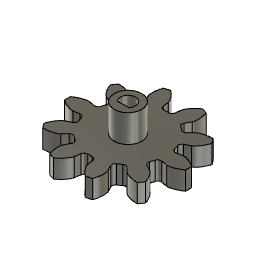
gear motor (Autodesk Fusion 360 design; units mm, degrees)
description: Spur Gear; Module: 2.2; Num Teeth: 10; Pressure Angle: 20.0; Backlash: 0.00 mm
Autodesk Fusion 360 part; units mm, degrees
(part 1 of 2)
sketch "gear motor 1" plane through (0, 0, 0) normal (0, 0, 1) x (1, 0, 0) in component "gear motor (1)"
  circle A0 centre (0, 0) radius 8.3092
  circle A1 centre (0, 0) radius 1.65
extrude "Extrude1" add sketch "gear motor 1" along normal blind 4 in component "gear motor (1)"
sketch "gear motor 2" plane through (0, 0, 0) normal (0, 0, 1) x (1, 0, 0) in component "gear motor (1)"
  spline S0 degree 5 poles (10.1841, -1.769) (10.1925, -1.7704) (10.2094, -1.7731) (10.2348, -1.7761) (10.2689, -1.7786) (10.3116, -1.7794) (10.3546, -1.7786) (10.3977, -1.7768) (10.4408, -1.7744) (10.484, -1.7717) (10.5273, -1.7685) (10.5706, -1.7648) (10.614, -1.7604) (10.6574, -1.7552) (10.7008, -1.7492) (10.7443, -1.7425) (10.7879, -1.7351) (10.8314, -1.7271) (10.875, -1.7187) (10.9186, -1.7098) (10.9622, -1.7005) (11.0058, -1.6907) (11.0494, -1.6804) (11.0931, -1.6695) (11.1367, -1.6581) (11.1803, -1.6463) (11.2239, -1.6339) (11.2675, -1.6212) (11.3111, -1.608) (11.3547, -1.5943) (11.3982, -1.5802) (11.4418, -1.5657) (11.4853, -1.5508) (11.5288, -1.5355) (11.5722, -1.5197) (11.6157, -1.5035) (11.6591, -1.4869) (11.7024, -1.4699) (11.7457, -1.4525) (11.789, -1.4347) (11.8323, -1.4166) (11.8755, -1.398) (11.9187, -1.3791) (11.9618, -1.3598) (12.0049, -1.3401) (12.0479, -1.32) (12.0909, -1.2996) (12.1338, -1.2787) (12.1766, -1.2576) (12.2194, -1.236) (12.2622, -1.2141) (12.3049, -1.1919) (12.3475, -1.1693) (12.3901, -1.1463) (12.4325, -1.123) (12.475, -1.0994) (12.5173, -1.0754) (12.5596, -1.0511) (12.6018, -1.0264) (12.6439, -1.0014) (12.686, -0.976) (12.728, -0.9503) (12.7699, -0.9243) (12.8117, -0.898) (12.8535, -0.8713) (12.8951, -0.8443) (12.9367, -0.817) (12.9782, -0.7893) (13.0195, -0.7613) (13.0608, -0.7331) (13.102, -0.7045) (13.1349, -0.6813) (13.1596, -0.6638) (13.176, -0.6521) (13.1842, -0.6462) knots 0 0 0 0 0 0 0.01428571 0.02857143 0.04285714 0.05714286 0.07142857 0.08571429 0.1 0.11428571 0.12857143 0.14285714 0.15714286 0.17142857 0.18571429 0.2 0.21428571 0.22857143 0.24285714 0.25714286 0.27142857 0.28571429 0.3 0.31428571 0.32857143 0.34285714 0.35714286 0.37142857 0.38571429 0.4 0.41428571 0.42857143 0.44285714 0.45714286 0.47142857 0.48571429 0.5 0.51428571 0.52857143 0.54285714 0.55714286 0.57142857 0.58571429 0.6 0.61428571 0.62857143 0.64285714 0.65714286 0.67142857 0.68571429 0.7 0.71428571 0.72857143 0.74285714 0.75714286 0.77142857 0.78571429 0.8 0.81428571 0.82857143 0.84285714 0.85714286 0.87142857 0.88571429 0.9 0.91428571 0.92857143 0.94285714 0.95714286 0.97142857 0.98571429 1 1 1 1 1 1
  spline S1 degree 5 poles (10.1841, 1.769) (10.1925, 1.7704) (10.2094, 1.7731) (10.2348, 1.7761) (10.2689, 1.7786) (10.3116, 1.7794) (10.3546, 1.7786) (10.3977, 1.7768) (10.4408, 1.7744) (10.484, 1.7717) (10.5273, 1.7685) (10.5706, 1.7648) (10.614, 1.7604) (10.6574, 1.7552) (10.7008, 1.7492) (10.7443, 1.7425) (10.7879, 1.7351) (10.8314, 1.7271) (10.875, 1.7187) (10.9186, 1.7098) (10.9622, 1.7005) (11.0058, 1.6907) (11.0494, 1.6804) (11.0931, 1.6695) (11.1367, 1.6581) (11.1803, 1.6463) (11.2239, 1.6339) (11.2675, 1.6212) (11.3111, 1.608) (11.3547, 1.5943) (11.3982, 1.5802) (11.4418, 1.5657) (11.4853, 1.5508) (11.5288, 1.5355) (11.5722, 1.5197) (11.6157, 1.5035) (11.6591, 1.4869) (11.7024, 1.4699) (11.7457, 1.4525) (11.789, 1.4347) (11.8323, 1.4166) (11.8755, 1.398) (11.9187, 1.3791) (11.9618, 1.3598) (12.0049, 1.3401) (12.0479, 1.32) (12.0909, 1.2996) (12.1338, 1.2787) (12.1766, 1.2576) (12.2194, 1.236) (12.2622, 1.2141) (12.3049, 1.1919) (12.3475, 1.1693) (12.3901, 1.1463) (12.4325, 1.123) (12.475, 1.0994) (12.5173, 1.0754) (12.5596, 1.0511) (12.6018, 1.0264) (12.6439, 1.0014) (12.686, 0.976) (12.728, 0.9503) (12.7699, 0.9243) (12.8117, 0.898) (12.8535, 0.8713) (12.8951, 0.8443) (12.9367, 0.817) (12.9782, 0.7893) (13.0195, 0.7613) (13.0608, 0.7331) (13.102, 0.7045) (13.1349, 0.6813) (13.1596, 0.6638) (13.176, 0.6521) (13.1842, 0.6462) knots 0 0 0 0 0 0 0.01428571 0.02857143 0.04285714 0.05714286 0.07142857 0.08571429 0.1 0.11428571 0.12857143 0.14285714 0.15714286 0.17142857 0.18571429 0.2 0.21428571 0.22857143 0.24285714 0.25714286 0.27142857 0.28571429 0.3 0.31428571 0.32857143 0.34285714 0.35714286 0.37142857 0.38571429 0.4 0.41428571 0.42857143 0.44285714 0.45714286 0.47142857 0.48571429 0.5 0.51428571 0.52857143 0.54285714 0.55714286 0.57142857 0.58571429 0.6 0.61428571 0.62857143 0.64285714 0.65714286 0.67142857 0.68571429 0.7 0.71428571 0.72857143 0.74285714 0.75714286 0.77142857 0.78571429 0.8 0.81428571 0.82857143 0.84285714 0.85714286 0.87142857 0.88571429 0.9 0.91428571 0.92857143 0.94285714 0.95714286 0.97142857 0.98571429 1 1 1 1 1 1
  arc A0 (13.1842, -0.6462) -> (13.1842, 0.6462) centre (0, 0) ccw
  line L0 (8.1768, -1.422) -> (10.1841, -1.769)
  line L1 (8.1768, 1.422) -> (10.1841, 1.769)
  line L2 (8.1768, -1.422) -> (8.1768, 1.422)
  point P0 (10.3903, -1.777)
  point P1 (10.6003, -1.7617)
  point P2 (10.8126, -1.7305)
  point P3 (11.0266, -1.6857)
  point P4 (11.2419, -1.6286)
  point P5 (11.4581, -1.5601)
  point P6 (11.6748, -1.4807)
  point P7 (11.8918, -1.3908)
  point P8 (12.1088, -1.2908)
  point P9 (12.3254, -1.1809)
  point P10 (12.5416, -1.0614)
  point P11 (12.7569, -0.9323)
  point P12 (12.9712, -0.7939)
  point P13 (10.3903, 1.777)
  point P14 (10.6003, 1.7617)
  point P15 (10.8126, 1.7305)
  point P16 (11.0266, 1.6857)
  point P17 (11.2419, 1.6286)
  point P18 (11.4581, 1.5601)
  point P19 (11.6748, 1.4807)
  point P20 (11.8918, 1.3908)
  point P21 (12.1088, 1.2908)
  point P22 (12.3254, 1.1809)
  point P23 (12.5416, 1.0614)
  point P24 (12.7569, 0.9323)
  point P25 (12.9712, 0.7939)
extrude "Extrude2" add sketch "gear motor 2" along normal blind 4 in component "gear motor (1)"
fillet "Fillet1" radius 0.75 2 edges at (8.1863, -1.4237, 2) (8.1863, 1.4237, 2) in component "gear motor (1)"
pattern_circular "C-Pattern1" count 10 over 360 about axis through (0, 0, 0) along (0, 0, 1) of "Extrude2", "Fillet1" in component "gear motor (1)"
sketch "gear motor 3" plane through (0, 0, 0) normal (0, 0, 1) x (1, 0, 0) in component "gear motor (1)"
  circle A0 centre (0, 0) radius 11 construction
mesh "Mesh1" [no effect] in component "gear motor (1)"
sketch "gear motor detailed cut" plane through (0, 0, 4) normal (0, 0, 1) x (-1, 0, 0) in component "gear motor (1)"
  arc A0 (-7.7368, 3.0305) -> (-8.0405, 2.0959) centre (0, 0) ccw
  arc A1 (-8.894, 1.546) -> (-8.0405, 2.0959) centre (-8.7663, 2.285) ccw
  line L0 (-8.894, 1.546) -> (-10.1841, 1.769)
  spline S0 degree 5 poles (-10.1841, 1.769) (-10.1925, 1.7704) (-10.2094, 1.7731) (-10.2348, 1.7761) (-10.2689, 1.7786) (-10.3116, 1.7794) (-10.3546, 1.7786) (-10.3977, 1.7768) (-10.4408, 1.7744) (-10.484, 1.7717) (-10.5273, 1.7685) (-10.5706, 1.7648) (-10.614, 1.7604) (-10.6574, 1.7552) (-10.7008, 1.7492) (-10.7443, 1.7425) (-10.7879, 1.7351) (-10.8314, 1.7271) (-10.875, 1.7187) (-10.9186, 1.7098) (-10.9622, 1.7005) (-11.0058, 1.6907) (-11.0494, 1.6804) (-11.0931, 1.6695) (-11.1367, 1.6581) (-11.1803, 1.6463) (-11.2239, 1.6339) (-11.2675, 1.6212) (-11.3111, 1.608) (-11.3547, 1.5943) (-11.3982, 1.5802) (-11.4418, 1.5657) (-11.4853, 1.5508) (-11.5288, 1.5355) (-11.5722, 1.5197) (-11.6157, 1.5035) (-11.6591, 1.4869) (-11.7024, 1.4699) (-11.7457, 1.4525) (-11.789, 1.4347) (-11.8323, 1.4166) (-11.8755, 1.398) (-11.9187, 1.3791) (-11.9618, 1.3598) (-12.0049, 1.3401) (-12.0479, 1.32) (-12.0909, 1.2996) (-12.1338, 1.2787) (-12.1766, 1.2576) (-12.2194, 1.236) (-12.2622, 1.2141) (-12.3049, 1.1919) (-12.3475, 1.1693) (-12.3901, 1.1463) (-12.4325, 1.123) (-12.475, 1.0994) (-12.5173, 1.0754) (-12.5596, 1.0511) (-12.6018, 1.0264) (-12.6439, 1.0014) (-12.686, 0.976) (-12.728, 0.9503) (-12.7699, 0.9243) (-12.8117, 0.898) (-12.8535, 0.8713) (-12.8951, 0.8443) (-12.9367, 0.817) (-12.9782, 0.7893) (-13.0195, 0.7613) (-13.0608, 0.7331) (-13.102, 0.7045) (-13.1349, 0.6813) (-13.1596, 0.6638) (-13.176, 0.6521) (-13.1842, 0.6462) knots 0 0 0 0 0 0 0.01428571 0.02857143 0.04285714 0.05714286 0.07142857 0.08571429 0.1 0.11428571 0.12857143 0.14285714 0.15714286 0.17142857 0.18571429 0.2 0.21428571 0.22857143 0.24285714 0.25714286 0.27142857 0.28571429 0.3 0.31428571 0.32857143 0.34285714 0.35714286 0.37142857 0.38571429 0.4 0.41428571 0.42857143 0.44285714 0.45714286 0.47142857 0.48571429 0.5 0.51428571 0.52857143 0.54285714 0.55714286 0.57142857 0.58571429 0.6 0.61428571 0.62857143 0.64285714 0.65714286 0.67142857 0.68571429 0.7 0.71428571 0.72857143 0.74285714 0.75714286 0.77142857 0.78571429 0.8 0.81428571 0.82857143 0.84285714 0.85714286 0.87142857 0.88571429 0.9 0.91428571 0.92857143 0.94285714 0.95714286 0.97142857 0.98571429 1 1 1 1 1 1
  arc A2 (-13.1842, 0.6462) -> (-13.1842, -0.6462) centre (0, 0) ccw
  spline S1 degree 5 poles (-13.1842, -0.6462) (-13.176, -0.6521) (-13.1596, -0.6638) (-13.1349, -0.6813) (-13.102, -0.7045) (-13.0608, -0.7331) (-13.0195, -0.7613) (-12.9782, -0.7893) (-12.9367, -0.817) (-12.8951, -0.8443) (-12.8535, -0.8713) (-12.8117, -0.898) (-12.7699, -0.9243) (-12.728, -0.9503) (-12.686, -0.976) (-12.6439, -1.0014) (-12.6018, -1.0264) (-12.5596, -1.0511) (-12.5173, -1.0754) (-12.475, -1.0994) (-12.4325, -1.123) (-12.3901, -1.1463) (-12.3475, -1.1693) (-12.3049, -1.1919) (-12.2622, -1.2141) (-12.2194, -1.236) (-12.1766, -1.2576) (-12.1338, -1.2787) (-12.0909, -1.2996) (-12.0479, -1.32) (-12.0049, -1.3401) (-11.9618, -1.3598) (-11.9187, -1.3791) (-11.8755, -1.398) (-11.8323, -1.4166) (-11.789, -1.4347) (-11.7457, -1.4525) (-11.7024, -1.4699) (-11.6591, -1.4869) (-11.6157, -1.5035) (-11.5722, -1.5197) (-11.5288, -1.5355) (-11.4853, -1.5508) (-11.4418, -1.5657) (-11.3982, -1.5802) (-11.3547, -1.5943) (-11.3111, -1.608) (-11.2675, -1.6212) (-11.2239, -1.6339) (-11.1803, -1.6463) (-11.1367, -1.6581) (-11.0931, -1.6695) (-11.0494, -1.6804) (-11.0058, -1.6907) (-10.9622, -1.7005) (-10.9186, -1.7098) (-10.875, -1.7187) (-10.8314, -1.7271) (-10.7879, -1.7351) (-10.7443, -1.7425) (-10.7008, -1.7492) (-10.6574, -1.7552) (-10.614, -1.7604) (-10.5706, -1.7648) (-10.5273, -1.7685) (-10.484, -1.7717) (-10.4408, -1.7744) (-10.3977, -1.7768) (-10.3546, -1.7786) (-10.3116, -1.7794) (-10.2689, -1.7786) (-10.2348, -1.7761) (-10.2094, -1.7731) (-10.1925, -1.7704) (-10.1841, -1.769) knots -1 -1 -1 -1 -1 -1 -0.98571429 -0.97142857 -0.95714286 -0.94285714 -0.92857143 -0.91428571 -0.9 -0.88571429 -0.87142857 -0.85714286 -0.84285714 -0.82857143 -0.81428571 -0.8 -0.78571429 -0.77142857 -0.75714286 -0.74285714 -0.72857143 -0.71428571 -0.7 -0.68571429 -0.67142857 -0.65714286 -0.64285714 -0.62857143 -0.61428571 -0.6 -0.58571429 -0.57142857 -0.55714286 -0.54285714 -0.52857143 -0.51428571 -0.5 -0.48571429 -0.47142857 -0.45714286 -0.44285714 -0.42857143 -0.41428571 -0.4 -0.38571429 -0.37142857 -0.35714286 -0.34285714 -0.32857143 -0.31428571 -0.3 -0.28571429 -0.27142857 -0.25714286 -0.24285714 -0.22857143 -0.21428571 -0.2 -0.18571429 -0.17142857 -0.15714286 -0.14285714 -0.12857143 -0.11428571 -0.1 -0.08571429 -0.07142857 -0.05714286 -0.04285714 -0.02857143 -0.01428571 0 0 0 0 0 0
  line L1 (-10.1841, -1.769) -> (-8.894, -1.546)
  arc A3 (-8.0405, -2.0959) -> (-8.894, -1.546) centre (-8.7663, -2.285) ccw
  arc A4 (-8.0405, -2.0959) -> (-7.7368, -3.0305) centre (0, 0) ccw
  arc A5 (-8.1041, -3.977) -> (-7.7368, -3.0305) centre (-8.4352, -3.3041) ccw
  line L2 (-8.1041, -3.977) -> (-9.2789, -4.5549)
  spline S2 degree 5 poles (-9.2789, -4.5549) (-9.2866, -4.5587) (-9.3018, -4.5665) (-9.3241, -4.579) (-9.3531, -4.597) (-9.3882, -4.6215) (-9.4225, -4.6474) (-9.4563, -4.6742) (-9.4898, -4.7014) (-9.5231, -4.7291) (-9.5563, -4.757) (-9.5891, -4.7855) (-9.6216, -4.8145) (-9.6537, -4.8442) (-9.6853, -4.8746) (-9.7166, -4.9057) (-9.7474, -4.9373) (-9.778, -4.9693) (-9.8083, -5.0017) (-9.8384, -5.0345) (-9.8682, -5.0677) (-9.8977, -5.1013) (-9.9269, -5.1353) (-9.9558, -5.1697) (-9.9844, -5.2045) (-10.0127, -5.2397) (-10.0407, -5.2754) (-10.0685, -5.3113) (-10.096, -5.3476) (-10.1232, -5.3843) (-10.1502, -5.4213) (-10.1769, -5.4586) (-10.2033, -5.4962) (-10.2295, -5.5342) (-10.2554, -5.5725) (-10.281, -5.6111) (-10.3064, -5.6501) (-10.3314, -5.6893) (-10.3563, -5.7289) (-10.3809, -5.7687) (-10.4052, -5.8088) (-10.4292, -5.8492) (-10.453, -5.8899) (-10.4765, -5.9309) (-10.4998, -5.9721) (-10.5228, -6.0137) (-10.5456, -6.0555) (-10.5681, -6.0975) (-10.5903, -6.1399) (-10.6123, -6.1824) (-10.634, -6.2253) (-10.6554, -6.2684) (-10.6766, -6.3117) (-10.6976, -6.3553) (-10.7182, -6.3991) (-10.7387, -6.4432) (-10.7588, -6.4875) (-10.7787, -6.532) (-10.7984, -6.5768) (-10.8178, -6.6218) (-10.8369, -6.667) (-10.8557, -6.7125) (-10.8744, -6.7582) (-10.8927, -6.8041) (-10.9108, -6.8502) (-10.9286, -6.8965) (-10.9462, -6.943) (-10.9635, -6.9898) (-10.9805, -7.0367) (-10.9973, -7.0839) (-11.0139, -7.1313) (-11.0269, -7.1693) (-11.0365, -7.198) (-11.0429, -7.2171) (-11.0461, -7.2267) knots 0 0 0 0 0 0 0.01428571 0.02857143 0.04285714 0.05714286 0.07142857 0.08571429 0.1 0.11428571 0.12857143 0.14285714 0.15714286 0.17142857 0.18571429 0.2 0.21428571 0.22857143 0.24285714 0.25714286 0.27142857 0.28571429 0.3 0.31428571 0.32857143 0.34285714 0.35714286 0.37142857 0.38571429 0.4 0.41428571 0.42857143 0.44285714 0.45714286 0.47142857 0.48571429 0.5 0.51428571 0.52857143 0.54285714 0.55714286 0.57142857 0.58571429 0.6 0.61428571 0.62857143 0.64285714 0.65714286 0.67142857 0.68571429 0.7 0.71428571 0.72857143 0.74285714 0.75714286 0.77142857 0.78571429 0.8 0.81428571 0.82857143 0.84285714 0.85714286 0.87142857 0.88571429 0.9 0.91428571 0.92857143 0.94285714 0.95714286 0.97142857 0.98571429 1 1 1 1 1 1
  arc A6 (-11.0461, -7.2267) -> (-10.2864, -8.2723) centre (0, 0) ccw
  spline S3 degree 5 poles (-10.2864, -8.2723) (-10.2763, -8.2722) (-10.2561, -8.2721) (-10.2259, -8.2717) (-10.1857, -8.2711) (-10.1356, -8.27) (-10.0855, -8.2686) (-10.0356, -8.2669) (-9.9858, -8.2649) (-9.9361, -8.2626) (-9.8865, -8.26) (-9.8371, -8.257) (-9.7878, -8.2537) (-9.7386, -8.2502) (-9.6895, -8.2463) (-9.6406, -8.242) (-9.5918, -8.2375) (-9.5431, -8.2327) (-9.4946, -8.2275) (-9.4463, -8.222) (-9.398, -8.2162) (-9.35, -8.2101) (-9.302, -8.2037) (-9.2543, -8.1969) (-9.2067, -8.1898) (-9.1592, -8.1824) (-9.1119, -8.1746) (-9.0648, -8.1666) (-9.0179, -8.1582) (-8.9711, -8.1495) (-8.9245, -8.1404) (-8.878, -8.131) (-8.8318, -8.1213) (-8.7858, -8.1113) (-8.7399, -8.1009) (-8.6942, -8.0902) (-8.6487, -8.0791) (-8.6035, -8.0677) (-8.5584, -8.056) (-8.5135, -8.0439) (-8.4689, -8.0314) (-8.4244, -8.0187) (-8.3802, -8.0055) (-8.3363, -7.992) (-8.2925, -7.9781) (-8.249, -7.9639) (-8.2057, -7.9494) (-8.1627, -7.9344) (-8.1199, -7.9191) (-8.0774, -7.9035) (-8.0351, -7.8874) (-7.9932, -7.871) (-7.9515, -7.8541) (-7.9101, -7.8369) (-7.8691, -7.8192) (-7.8283, -7.8011) (-7.7879, -7.7826) (-7.7476, -7.7638) (-7.7077, -7.7447) (-7.6682, -7.7251) (-7.629, -7.7049) (-7.5903, -7.6843) (-7.5521, -7.663) (-7.5144, -7.641) (-7.4772, -7.6186) (-7.4404, -7.5957) (-7.4038, -7.5725) (-7.3675, -7.549) (-7.3316, -7.5252) (-7.2964, -7.5006) (-7.2623, -7.4748) (-7.2362, -7.4528) (-7.2174, -7.4354) (-7.2053, -7.4233) (-7.1993, -7.4172) knots -1 -1 -1 -1 -1 -1 -0.98571429 -0.97142857 -0.95714286 -0.94285714 -0.92857143 -0.91428571 -0.9 -0.88571429 -0.87142857 -0.85714286 -0.84285714 -0.82857143 -0.81428571 -0.8 -0.78571429 -0.77142857 -0.75714286 -0.74285714 -0.72857143 -0.71428571 -0.7 -0.68571429 -0.67142857 -0.65714286 -0.64285714 -0.62857143 -0.61428571 -0.6 -0.58571429 -0.57142857 -0.55714286 -0.54285714 -0.52857143 -0.51428571 -0.5 -0.48571429 -0.47142857 -0.45714286 -0.44285714 -0.42857143 -0.41428571 -0.4 -0.38571429 -0.37142857 -0.35714286 -0.34285714 -0.32857143 -0.31428571 -0.3 -0.28571429 -0.27142857 -0.25714286 -0.24285714 -0.22857143 -0.21428571 -0.2 -0.18571429 -0.17142857 -0.15714286 -0.14285714 -0.12857143 -0.11428571 -0.1 -0.08571429 -0.07142857 -0.05714286 -0.04285714 -0.02857143 -0.01428571 0 0 0 0 0 0
  line L3 (-7.1993, -7.4172) -> (-6.2867, -6.4785)
  arc A7 (-5.273, -6.4217) -> (-6.2867, -6.4785) centre (-5.749, -7.0013) ccw
  arc A8 (-5.273, -6.4217) -> (-4.4779, -6.9993) centre (0, 0) ccw
  arc A9 (-4.2187, -7.981) -> (-4.4779, -6.9993) centre (-4.8821, -7.6311) ccw
  line L4 (-4.2187, -7.981) -> (-4.8295, -9.139)
  spline S4 degree 5 poles (-4.8295, -9.139) (-4.8335, -9.1466) (-4.8412, -9.1618) (-4.8519, -9.185) (-4.8648, -9.2167) (-4.8788, -9.2571) (-4.8913, -9.2982) (-4.9029, -9.3397) (-4.914, -9.3815) (-4.9247, -9.4234) (-4.9351, -9.4655) (-4.945, -9.5079) (-4.9542, -9.5505) (-4.9626, -9.5934) (-4.9704, -9.6366) (-4.9774, -9.68) (-4.9838, -9.7237) (-4.9897, -9.7676) (-4.9952, -9.8117) (-5.0002, -9.8559) (-5.0048, -9.9002) (-5.0089, -9.9447) (-5.0126, -9.9894) (-5.0157, -10.0342) (-5.0184, -10.0792) (-5.0206, -10.1244) (-5.0224, -10.1697) (-5.0237, -10.2151) (-5.0246, -10.2606) (-5.0251, -10.3063) (-5.0251, -10.352) (-5.0248, -10.3979) (-5.0241, -10.4439) (-5.0229, -10.49) (-5.0213, -10.5362) (-5.0194, -10.5825) (-5.017, -10.6289) (-5.0142, -10.6754) (-5.0111, -10.722) (-5.0075, -10.7687) (-5.0036, -10.8154) (-4.9993, -10.8623) (-4.9947, -10.9092) (-4.9896, -10.9562) (-4.9842, -11.0032) (-4.9784, -11.0503) (-4.9722, -11.0975) (-4.9657, -11.1448) (-4.9588, -11.1921) (-4.9516, -11.2394) (-4.9439, -11.2868) (-4.936, -11.3343) (-4.9277, -11.3818) (-4.919, -11.4294) (-4.9099, -11.477) (-4.9006, -11.5247) (-4.8908, -11.5724) (-4.8807, -11.6201) (-4.8703, -11.6679) (-4.8595, -11.7157) (-4.8484, -11.7635) (-4.837, -11.8114) (-4.8252, -11.8593) (-4.8131, -11.9072) (-4.8006, -11.9551) (-4.7878, -12.0031) (-4.7746, -12.0511) (-4.7612, -12.099) (-4.7473, -12.1471) (-4.7332, -12.1951) (-4.7187, -12.2431) (-4.7069, -12.2815) (-4.6979, -12.3104) (-4.6918, -12.3296) (-4.6887, -12.3392) knots 0 0 0 0 0 0 0.01428571 0.02857143 0.04285714 0.05714286 0.07142857 0.08571429 0.1 0.11428571 0.12857143 0.14285714 0.15714286 0.17142857 0.18571429 0.2 0.21428571 0.22857143 0.24285714 0.25714286 0.27142857 0.28571429 0.3 0.31428571 0.32857143 0.34285714 0.35714286 0.37142857 0.38571429 0.4 0.41428571 0.42857143 0.44285714 0.45714286 0.47142857 0.48571429 0.5 0.51428571 0.52857143 0.54285714 0.55714286 0.57142857 0.58571429 0.6 0.61428571 0.62857143 0.64285714 0.65714286 0.67142857 0.68571429 0.7 0.71428571 0.72857143 0.74285714 0.75714286 0.77142857 0.78571429 0.8 0.81428571 0.82857143 0.84285714 0.85714286 0.87142857 0.88571429 0.9 0.91428571 0.92857143 0.94285714 0.95714286 0.97142857 0.98571429 1 1 1 1 1 1
  arc A10 (-4.6887, -12.3392) -> (-3.4595, -12.7386) centre (0, 0) ccw
  spline S5 degree 5 poles (-3.4595, -12.7386) (-3.4514, -12.7326) (-3.4352, -12.7206) (-3.4109, -12.7026) (-3.3788, -12.6785) (-3.3388, -12.6481) (-3.2992, -12.6176) (-3.2598, -12.5869) (-3.2207, -12.556) (-3.1818, -12.5249) (-3.1433, -12.4936) (-3.105, -12.4621) (-3.067, -12.4305) (-3.0293, -12.3987) (-2.9919, -12.3667) (-2.9548, -12.3345) (-2.918, -12.3022) (-2.8815, -12.2697) (-2.8453, -12.237) (-2.8094, -12.2041) (-2.7738, -12.1711) (-2.7385, -12.1379) (-2.7035, -12.1045) (-2.6689, -12.0709) (-2.6345, -12.0372) (-2.6005, -12.0033) (-2.5668, -11.9693) (-2.5334, -11.9351) (-2.5003, -11.9007) (-2.4676, -11.8661) (-2.4352, -11.8314) (-2.4032, -11.7965) (-2.3715, -11.7615) (-2.3401, -11.7263) (-2.3091, -11.6909) (-2.2785, -11.6554) (-2.2482, -11.6197) (-2.2183, -11.5839) (-2.1887, -11.5479) (-2.1595, -11.5117) (-2.1307, -11.4754) (-2.1023, -11.439) (-2.0742, -11.4024) (-2.0466, -11.3656) (-2.0194, -11.3287) (-1.9925, -11.2916) (-1.9661, -11.2544) (-1.94, -11.217) (-1.9144, -11.1795) (-1.8892, -11.1418) (-1.8644, -11.104) (-1.8402, -11.066) (-1.8164, -11.0279) (-1.7931, -10.9896) (-1.7702, -10.9512) (-1.7479, -10.9126) (-1.726, -10.8739) (-1.7045, -10.835) (-1.6835, -10.7961) (-1.663, -10.7569) (-1.6431, -10.7176) (-1.624, -10.6782) (-1.6056, -10.6385) (-1.588, -10.5986) (-1.5711, -10.5586) (-1.5548, -10.5184) (-1.5388, -10.4781) (-1.5233, -10.4378) (-1.5082, -10.3974) (-1.4942, -10.3568) (-1.4817, -10.3159) (-1.4735, -10.2827) (-1.4686, -10.2576) (-1.4659, -10.2408) (-1.4647, -10.2323) knots -1 -1 -1 -1 -1 -1 -0.98571429 -0.97142857 -0.95714286 -0.94285714 -0.92857143 -0.91428571 -0.9 -0.88571429 -0.87142857 -0.85714286 -0.84285714 -0.82857143 -0.81428571 -0.8 -0.78571429 -0.77142857 -0.75714286 -0.74285714 -0.72857143 -0.71428571 -0.7 -0.68571429 -0.67142857 -0.65714286 -0.64285714 -0.62857143 -0.61428571 -0.6 -0.58571429 -0.57142857 -0.55714286 -0.54285714 -0.52857143 -0.51428571 -0.5 -0.48571429 -0.47142857 -0.45714286 -0.44285714 -0.42857143 -0.41428571 -0.4 -0.38571429 -0.37142857 -0.35714286 -0.34285714 -0.32857143 -0.31428571 -0.3 -0.28571429 -0.27142857 -0.25714286 -0.24285714 -0.22857143 -0.21428571 -0.2 -0.18571429 -0.17142857 -0.15714286 -0.14285714 -0.12857143 -0.11428571 -0.1 -0.08571429 -0.07142857 -0.05714286 -0.04285714 -0.02857143 -0.01428571 0 0 0 0 0 0
  line L5 (-1.4647, -10.2323) -> (-1.2781, -8.9365)
  arc A11 (-0.4914, -8.2947) -> (-1.2781, -8.9365) centre (-0.5357, -9.0433) ccw
  arc A12 (-0.4914, -8.2947) -> (0.4914, -8.2947) centre (0, 0) ccw
  arc A13 (1.2781, -8.9365) -> (0.4914, -8.2947) centre (0.5357, -9.0433) ccw
  line L6 (1.2781, -8.9365) -> (1.4647, -10.2323)
  spline S6 degree 5 poles (1.4647, -10.2323) (1.4659, -10.2408) (1.4686, -10.2576) (1.4735, -10.2827) (1.4817, -10.3159) (1.4942, -10.3568) (1.5082, -10.3974) (1.5233, -10.4378) (1.5388, -10.4781) (1.5548, -10.5184) (1.5711, -10.5586) (1.588, -10.5986) (1.6056, -10.6385) (1.624, -10.6782) (1.6431, -10.7176) (1.663, -10.7569) (1.6835, -10.7961) (1.7045, -10.835) (1.726, -10.8739) (1.7479, -10.9126) (1.7702, -10.9512) (1.7931, -10.9896) (1.8164, -11.0279) (1.8402, -11.066) (1.8644, -11.104) (1.8892, -11.1418) (1.9144, -11.1795) (1.94, -11.217) (1.9661, -11.2544) (1.9925, -11.2916) (2.0194, -11.3287) (2.0466, -11.3656) (2.0742, -11.4024) (2.1023, -11.439) (2.1307, -11.4754) (2.1595, -11.5117) (2.1887, -11.5479) (2.2183, -11.5839) (2.2482, -11.6197) (2.2785, -11.6554) (2.3091, -11.6909) (2.3401, -11.7263) (2.3715, -11.7615) (2.4032, -11.7965) (2.4352, -11.8314) (2.4676, -11.8661) (2.5003, -11.9007) (2.5334, -11.9351) (2.5668, -11.9693) (2.6005, -12.0033) (2.6345, -12.0372) (2.6689, -12.0709) (2.7035, -12.1045) (2.7385, -12.1379) (2.7738, -12.1711) (2.8094, -12.2041) (2.8453, -12.237) (2.8815, -12.2697) (2.918, -12.3022) (2.9548, -12.3345) (2.9919, -12.3667) (3.0293, -12.3987) (3.067, -12.4305) (3.105, -12.4621) (3.1433, -12.4936) (3.1818, -12.5249) (3.2207, -12.556) (3.2598, -12.5869) (3.2992, -12.6176) (3.3388, -12.6481) (3.3788, -12.6785) (3.4109, -12.7026) (3.4352, -12.7206) (3.4514, -12.7326) (3.4595, -12.7386) knots 0 0 0 0 0 0 0.01428571 0.02857143 0.04285714 0.05714286 0.07142857 0.08571429 0.1 0.11428571 0.12857143 0.14285714 0.15714286 0.17142857 0.18571429 0.2 0.21428571 0.22857143 0.24285714 0.25714286 0.27142857 0.28571429 0.3 0.31428571 0.32857143 0.34285714 0.35714286 0.37142857 0.38571429 0.4 0.41428571 0.42857143 0.44285714 0.45714286 0.47142857 0.48571429 0.5 0.51428571 0.52857143 0.54285714 0.55714286 0.57142857 0.58571429 0.6 0.61428571 0.62857143 0.64285714 0.65714286 0.67142857 0.68571429 0.7 0.71428571 0.72857143 0.74285714 0.75714286 0.77142857 0.78571429 0.8 0.81428571 0.82857143 0.84285714 0.85714286 0.87142857 0.88571429 0.9 0.91428571 0.92857143 0.94285714 0.95714286 0.97142857 0.98571429 1 1 1 1 1 1
  arc A14 (3.4595, -12.7386) -> (4.6887, -12.3392) centre (0, 0) ccw
  spline S7 degree 5 poles (4.6887, -12.3392) (4.6918, -12.3296) (4.6979, -12.3104) (4.7069, -12.2815) (4.7187, -12.2431) (4.7332, -12.1951) (4.7473, -12.1471) (4.7612, -12.099) (4.7746, -12.0511) (4.7878, -12.0031) (4.8006, -11.9551) (4.8131, -11.9072) (4.8252, -11.8593) (4.837, -11.8114) (4.8484, -11.7635) (4.8595, -11.7157) (4.8703, -11.6679) (4.8807, -11.6201) (4.8908, -11.5724) (4.9006, -11.5247) (4.9099, -11.477) (4.919, -11.4294) (4.9277, -11.3818) (4.936, -11.3343) (4.9439, -11.2868) (4.9516, -11.2394) (4.9588, -11.1921) (4.9657, -11.1448) (4.9722, -11.0975) (4.9784, -11.0503) (4.9842, -11.0032) (4.9896, -10.9562) (4.9947, -10.9092) (4.9993, -10.8623) (5.0036, -10.8154) (5.0075, -10.7687) (5.0111, -10.722) (5.0142, -10.6754) (5.017, -10.6289) (5.0194, -10.5825) (5.0213, -10.5362) (5.0229, -10.49) (5.0241, -10.4439) (5.0248, -10.3979) (5.0251, -10.352) (5.0251, -10.3063) (5.0246, -10.2606) (5.0237, -10.2151) (5.0224, -10.1697) (5.0206, -10.1244) (5.0184, -10.0792) (5.0157, -10.0342) (5.0126, -9.9894) (5.0089, -9.9447) (5.0048, -9.9002) (5.0002, -9.8559) (4.9952, -9.8117) (4.9897, -9.7676) (4.9838, -9.7237) (4.9774, -9.68) (4.9704, -9.6366) (4.9626, -9.5934) (4.9542, -9.5505) (4.945, -9.5079) (4.9351, -9.4655) (4.9247, -9.4234) (4.914, -9.3815) (4.9029, -9.3397) (4.8913, -9.2982) (4.8788, -9.2571) (4.8648, -9.2167) (4.8519, -9.185) (4.8412, -9.1618) (4.8335, -9.1466) (4.8295, -9.139) knots -1 -1 -1 -1 -1 -1 -0.98571429 -0.97142857 -0.95714286 -0.94285714 -0.92857143 -0.91428571 -0.9 -0.88571429 -0.87142857 -0.85714286 -0.84285714 -0.82857143 -0.81428571 -0.8 -0.78571429 -0.77142857 -0.75714286 -0.74285714 -0.72857143 -0.71428571 -0.7 -0.68571429 -0.67142857 -0.65714286 -0.64285714 -0.62857143 -0.61428571 -0.6 -0.58571429 -0.57142857 -0.55714286 -0.54285714 -0.52857143 -0.51428571 -0.5 -0.48571429 -0.47142857 -0.45714286 -0.44285714 -0.42857143 -0.41428571 -0.4 -0.38571429 -0.37142857 -0.35714286 -0.34285714 -0.32857143 -0.31428571 -0.3 -0.28571429 -0.27142857 -0.25714286 -0.24285714 -0.22857143 -0.21428571 -0.2 -0.18571429 -0.17142857 -0.15714286 -0.14285714 -0.12857143 -0.11428571 -0.1 -0.08571429 -0.07142857 -0.05714286 -0.04285714 -0.02857143 -0.01428571 0 0 0 0 0 0
  line L7 (4.8295, -9.139) -> (4.2187, -7.981)
  arc A15 (4.4779, -6.9993) -> (4.2187, -7.981) centre (4.8821, -7.6311) ccw
  arc A16 (4.4779, -6.9993) -> (5.273, -6.4217) centre (0, 0) ccw
  arc A17 (6.2867, -6.4785) -> (5.273, -6.4217) centre (5.749, -7.0013) ccw
  line L8 (6.2867, -6.4785) -> (7.1993, -7.4172)
  spline S8 degree 5 poles (7.1993, -7.4172) (7.2053, -7.4233) (7.2174, -7.4354) (7.2362, -7.4528) (7.2623, -7.4748) (7.2964, -7.5006) (7.3316, -7.5252) (7.3675, -7.549) (7.4038, -7.5725) (7.4404, -7.5957) (7.4772, -7.6186) (7.5144, -7.641) (7.5521, -7.663) (7.5903, -7.6843) (7.629, -7.7049) (7.6682, -7.7251) (7.7077, -7.7447) (7.7476, -7.7638) (7.7879, -7.7826) (7.8283, -7.8011) (7.8691, -7.8192) (7.9101, -7.8369) (7.9515, -7.8541) (7.9932, -7.871) (8.0351, -7.8874) (8.0774, -7.9035) (8.1199, -7.9191) (8.1627, -7.9344) (8.2057, -7.9494) (8.249, -7.9639) (8.2925, -7.9781) (8.3363, -7.992) (8.3802, -8.0055) (8.4244, -8.0187) (8.4689, -8.0314) (8.5135, -8.0439) (8.5584, -8.056) (8.6035, -8.0677) (8.6487, -8.0791) (8.6942, -8.0902) (8.7399, -8.1009) (8.7858, -8.1113) (8.8318, -8.1213) (8.878, -8.131) (8.9245, -8.1404) (8.9711, -8.1495) (9.0179, -8.1582) (9.0648, -8.1666) (9.1119, -8.1746) (9.1592, -8.1824) (9.2067, -8.1898) (9.2543, -8.1969) (9.302, -8.2037) (9.35, -8.2101) (9.398, -8.2162) (9.4463, -8.222) (9.4946, -8.2275) (9.5431, -8.2327) (9.5918, -8.2375) (9.6406, -8.242) (9.6895, -8.2463) (9.7386, -8.2502) (9.7878, -8.2537) (9.8371, -8.257) (9.8865, -8.26) (9.9361, -8.2626) (9.9858, -8.2649) (10.0356, -8.2669) (10.0855, -8.2686) (10.1356, -8.27) (10.1857, -8.2711) (10.2259, -8.2717) (10.2561, -8.2721) (10.2763, -8.2722) (10.2864, -8.2723) knots 0 0 0 0 0 0 0.01428571 0.02857143 0.04285714 0.05714286 0.07142857 0.08571429 0.1 0.11428571 0.12857143 0.14285714 0.15714286 0.17142857 0.18571429 0.2 0.21428571 0.22857143 0.24285714 0.25714286 0.27142857 0.28571429 0.3 0.31428571 0.32857143 0.34285714 0.35714286 0.37142857 0.38571429 0.4 0.41428571 0.42857143 0.44285714 0.45714286 0.47142857 0.48571429 0.5 0.51428571 0.52857143 0.54285714 0.55714286 0.57142857 0.58571429 0.6 0.61428571 0.62857143 0.64285714 0.65714286 0.67142857 0.68571429 0.7 0.71428571 0.72857143 0.74285714 0.75714286 0.77142857 0.78571429 0.8 0.81428571 0.82857143 0.84285714 0.85714286 0.87142857 0.88571429 0.9 0.91428571 0.92857143 0.94285714 0.95714286 0.97142857 0.98571429 1 1 1 1 1 1
  arc A18 (10.2864, -8.2723) -> (11.0461, -7.2267) centre (0, 0) ccw
  spline S9 degree 5 poles (11.0461, -7.2267) (11.0429, -7.2171) (11.0365, -7.198) (11.0269, -7.1693) (11.0139, -7.1313) (10.9973, -7.0839) (10.9805, -7.0367) (10.9635, -6.9898) (10.9462, -6.943) (10.9286, -6.8965) (10.9108, -6.8502) (10.8927, -6.8041) (10.8744, -6.7582) (10.8557, -6.7125) (10.8369, -6.667) (10.8178, -6.6218) (10.7984, -6.5768) (10.7787, -6.532) (10.7588, -6.4875) (10.7387, -6.4432) (10.7182, -6.3991) (10.6976, -6.3553) (10.6766, -6.3117) (10.6554, -6.2684) (10.634, -6.2253) (10.6123, -6.1824) (10.5903, -6.1399) (10.5681, -6.0975) (10.5456, -6.0555) (10.5228, -6.0137) (10.4998, -5.9721) (10.4765, -5.9309) (10.453, -5.8899) (10.4292, -5.8492) (10.4052, -5.8088) (10.3809, -5.7687) (10.3563, -5.7289) (10.3314, -5.6893) (10.3064, -5.6501) (10.281, -5.6111) (10.2554, -5.5725) (10.2295, -5.5342) (10.2033, -5.4962) (10.1769, -5.4586) (10.1502, -5.4213) (10.1232, -5.3843) (10.096, -5.3476) (10.0685, -5.3113) (10.0407, -5.2754) (10.0127, -5.2397) (9.9844, -5.2045) (9.9558, -5.1697) (9.9269, -5.1353) (9.8977, -5.1013) (9.8682, -5.0677) (9.8384, -5.0345) (9.8083, -5.0017) (9.778, -4.9693) (9.7474, -4.9373) (9.7166, -4.9057) (9.6853, -4.8746) (9.6537, -4.8442) (9.6216, -4.8145) (9.5891, -4.7855) (9.5563, -4.757) (9.5231, -4.7291) (9.4898, -4.7014) (9.4563, -4.6742) (9.4225, -4.6474) (9.3882, -4.6215) (9.3531, -4.597) (9.3241, -4.579) (9.3018, -4.5665) (9.2866, -4.5587) (9.2789, -4.5549) knots -1 -1 -1 -1 -1 -1 -0.98571429 -0.97142857 -0.95714286 -0.94285714 -0.92857143 -0.91428571 -0.9 -0.88571429 -0.87142857 -0.85714286 -0.84285714 -0.82857143 -0.81428571 -0.8 -0.78571429 -0.77142857 -0.75714286 -0.74285714 -0.72857143 -0.71428571 -0.7 -0.68571429 -0.67142857 -0.65714286 -0.64285714 -0.62857143 -0.61428571 -0.6 -0.58571429 -0.57142857 -0.55714286 -0.54285714 -0.52857143 -0.51428571 -0.5 -0.48571429 -0.47142857 -0.45714286 -0.44285714 -0.42857143 -0.41428571 -0.4 -0.38571429 -0.37142857 -0.35714286 -0.34285714 -0.32857143 -0.31428571 -0.3 -0.28571429 -0.27142857 -0.25714286 -0.24285714 -0.22857143 -0.21428571 -0.2 -0.18571429 -0.17142857 -0.15714286 -0.14285714 -0.12857143 -0.11428571 -0.1 -0.08571429 -0.07142857 -0.05714286 -0.04285714 -0.02857143 -0.01428571 0 0 0 0 0 0
  line L9 (9.2789, -4.5549) -> (8.1041, -3.977)
  arc A19 (7.7368, -3.0305) -> (8.1041, -3.977) centre (8.4352, -3.3041) ccw
  arc A20 (7.7368, -3.0305) -> (8.0405, -2.0959) centre (0, 0) ccw
  arc A21 (8.894, -1.546) -> (8.0405, -2.0959) centre (8.7663, -2.285) ccw
  line L10 (8.894, -1.546) -> (10.1841, -1.769)
  spline S10 degree 5 poles (10.1841, -1.769) (10.1925, -1.7704) (10.2094, -1.7731) (10.2348, -1.7761) (10.2689, -1.7786) (10.3116, -1.7794) (10.3546, -1.7786) (10.3977, -1.7768) (10.4408, -1.7744) (10.484, -1.7717) (10.5273, -1.7685) (10.5706, -1.7648) (10.614, -1.7604) (10.6574, -1.7552) (10.7008, -1.7492) (10.7443, -1.7425) (10.7879, -1.7351) (10.8314, -1.7271) (10.875, -1.7187) (10.9186, -1.7098) (10.9622, -1.7005) (11.0058, -1.6907) (11.0494, -1.6804) (11.0931, -1.6695) (11.1367, -1.6581) (11.1803, -1.6463) (11.2239, -1.6339) (11.2675, -1.6212) (11.3111, -1.608) (11.3547, -1.5943) (11.3982, -1.5802) (11.4418, -1.5657) (11.4853, -1.5508) (11.5288, -1.5355) (11.5722, -1.5197) (11.6157, -1.5035) (11.6591, -1.4869) (11.7024, -1.4699) (11.7457, -1.4525) (11.789, -1.4347) (11.8323, -1.4166) (11.8755, -1.398) (11.9187, -1.3791) (11.9618, -1.3598) (12.0049, -1.3401) (12.0479, -1.32) (12.0909, -1.2996) (12.1338, -1.2787) (12.1766, -1.2576) (12.2194, -1.236) (12.2622, -1.2141) (12.3049, -1.1919) (12.3475, -1.1693) (12.3901, -1.1463) (12.4325, -1.123) (12.475, -1.0994) (12.5173, -1.0754) (12.5596, -1.0511) (12.6018, -1.0264) (12.6439, -1.0014) (12.686, -0.976) (12.728, -0.9503) (12.7699, -0.9243) (12.8117, -0.898) (12.8535, -0.8713) (12.8951, -0.8443) (12.9367, -0.817) (12.9782, -0.7893) (13.0195, -0.7613) (13.0608, -0.7331) (13.102, -0.7045) (13.1349, -0.6813) (13.1596, -0.6638) (13.176, -0.6521) (13.1842, -0.6462) knots 0 0 0 0 0 0 0.01428571 0.02857143 0.04285714 0.05714286 0.07142857 0.08571429 0.1 0.11428571 0.12857143 0.14285714 0.15714286 0.17142857 0.18571429 0.2 0.21428571 0.22857143 0.24285714 0.25714286 0.27142857 0.28571429 0.3 0.31428571 0.32857143 0.34285714 0.35714286 0.37142857 0.38571429 0.4 0.41428571 0.42857143 0.44285714 0.45714286 0.47142857 0.48571429 0.5 0.51428571 0.52857143 0.54285714 0.55714286 0.57142857 0.58571429 0.6 0.61428571 0.62857143 0.64285714 0.65714286 0.67142857 0.68571429 0.7 0.71428571 0.72857143 0.74285714 0.75714286 0.77142857 0.78571429 0.8 0.81428571 0.82857143 0.84285714 0.85714286 0.87142857 0.88571429 0.9 0.91428571 0.92857143 0.94285714 0.95714286 0.97142857 0.98571429 1 1 1 1 1 1
  arc A22 (13.1842, -0.6462) -> (13.1842, 0.6462) centre (0, 0) ccw
  spline S11 degree 5 poles (13.1842, 0.6462) (13.176, 0.6521) (13.1596, 0.6638) (13.1349, 0.6813) (13.102, 0.7045) (13.0608, 0.7331) (13.0195, 0.7613) (12.9782, 0.7893) (12.9367, 0.817) (12.8951, 0.8443) (12.8535, 0.8713) (12.8117, 0.898) (12.7699, 0.9243) (12.728, 0.9503) (12.686, 0.976) (12.6439, 1.0014) (12.6018, 1.0264) (12.5596, 1.0511) (12.5173, 1.0754) (12.475, 1.0994) (12.4325, 1.123) (12.3901, 1.1463) (12.3475, 1.1693) (12.3049, 1.1919) (12.2622, 1.2141) (12.2194, 1.236) (12.1766, 1.2576) (12.1338, 1.2787) (12.0909, 1.2996) (12.0479, 1.32) (12.0049, 1.3401) (11.9618, 1.3598) (11.9187, 1.3791) (11.8755, 1.398) (11.8323, 1.4166) (11.789, 1.4347) (11.7457, 1.4525) (11.7024, 1.4699) (11.6591, 1.4869) (11.6157, 1.5035) (11.5722, 1.5197) (11.5288, 1.5355) (11.4853, 1.5508) (11.4418, 1.5657) (11.3982, 1.5802) (11.3547, 1.5943) (11.3111, 1.608) (11.2675, 1.6212) (11.2239, 1.6339) (11.1803, 1.6463) (11.1367, 1.6581) (11.0931, 1.6695) (11.0494, 1.6804) (11.0058, 1.6907) (10.9622, 1.7005) (10.9186, 1.7098) (10.875, 1.7187) (10.8314, 1.7271) (10.7879, 1.7351) (10.7443, 1.7425) (10.7008, 1.7492) (10.6574, 1.7552) (10.614, 1.7604) (10.5706, 1.7648) (10.5273, 1.7685) (10.484, 1.7717) (10.4408, 1.7744) (10.3977, 1.7768) (10.3546, 1.7786) (10.3116, 1.7794) (10.2689, 1.7786) (10.2348, 1.7761) (10.2094, 1.7731) (10.1925, 1.7704) (10.1841, 1.769) knots -1 -1 -1 -1 -1 -1 -0.98571429 -0.97142857 -0.95714286 -0.94285714 -0.92857143 -0.91428571 -0.9 -0.88571429 -0.87142857 -0.85714286 -0.84285714 -0.82857143 -0.81428571 -0.8 -0.78571429 -0.77142857 -0.75714286 -0.74285714 -0.72857143 -0.71428571 -0.7 -0.68571429 -0.67142857 -0.65714286 -0.64285714 -0.62857143 -0.61428571 -0.6 -0.58571429 -0.57142857 -0.55714286 -0.54285714 -0.52857143 -0.51428571 -0.5 -0.48571429 -0.47142857 -0.45714286 -0.44285714 -0.42857143 -0.41428571 -0.4 -0.38571429 -0.37142857 -0.35714286 -0.34285714 -0.32857143 -0.31428571 -0.3 -0.28571429 -0.27142857 -0.25714286 -0.24285714 -0.22857143 -0.21428571 -0.2 -0.18571429 -0.17142857 -0.15714286 -0.14285714 -0.12857143 -0.11428571 -0.1 -0.08571429 -0.07142857 -0.05714286 -0.04285714 -0.02857143 -0.01428571 0 0 0 0 0 0
  line L11 (10.1841, 1.769) -> (8.894, 1.546)
  arc A23 (8.0405, 2.0959) -> (8.894, 1.546) centre (8.7663, 2.285) ccw
  arc A24 (8.0405, 2.0959) -> (7.7368, 3.0305) centre (0, 0) ccw
  arc A25 (8.1041, 3.977) -> (7.7368, 3.0305) centre (8.4352, 3.3041) ccw
  line L12 (8.1041, 3.977) -> (9.2789, 4.5549)
  spline S12 degree 5 poles (9.2789, 4.5549) (9.2866, 4.5587) (9.3018, 4.5665) (9.3241, 4.579) (9.3531, 4.597) (9.3882, 4.6215) (9.4225, 4.6474) (9.4563, 4.6742) (9.4898, 4.7014) (9.5231, 4.7291) (9.5563, 4.757) (9.5891, 4.7855) (9.6216, 4.8145) (9.6537, 4.8442) (9.6853, 4.8746) (9.7166, 4.9057) (9.7474, 4.9373) (9.778, 4.9693) (9.8083, 5.0017) (9.8384, 5.0345) (9.8682, 5.0677) (9.8977, 5.1013) (9.9269, 5.1353) (9.9558, 5.1697) (9.9844, 5.2045) (10.0127, 5.2397) (10.0407, 5.2754) (10.0685, 5.3113) (10.096, 5.3476) (10.1232, 5.3843) (10.1502, 5.4213) (10.1769, 5.4586) (10.2033, 5.4962) (10.2295, 5.5342) (10.2554, 5.5725) (10.281, 5.6111) (10.3064, 5.6501) (10.3314, 5.6893) (10.3563, 5.7289) (10.3809, 5.7687) (10.4052, 5.8088) (10.4292, 5.8492) (10.453, 5.8899) (10.4765, 5.9309) (10.4998, 5.9721) (10.5228, 6.0137) (10.5456, 6.0555) (10.5681, 6.0975) (10.5903, 6.1399) (10.6123, 6.1824) (10.634, 6.2253) (10.6554, 6.2684) (10.6766, 6.3117) (10.6976, 6.3553) (10.7182, 6.3991) (10.7387, 6.4432) (10.7588, 6.4875) (10.7787, 6.532) (10.7984, 6.5768) (10.8178, 6.6218) (10.8369, 6.667) (10.8557, 6.7125) (10.8744, 6.7582) (10.8927, 6.8041) (10.9108, 6.8502) (10.9286, 6.8965) (10.9462, 6.943) (10.9635, 6.9898) (10.9805, 7.0367) (10.9973, 7.0839) (11.0139, 7.1313) (11.0269, 7.1693) (11.0365, 7.198) (11.0429, 7.2171) (11.0461, 7.2267) knots 0 0 0 0 0 0 0.01428571 0.02857143 0.04285714 0.05714286 0.07142857 0.08571429 0.1 0.11428571 0.12857143 0.14285714 0.15714286 0.17142857 0.18571429 0.2 0.21428571 0.22857143 0.24285714 0.25714286 0.27142857 0.28571429 0.3 0.31428571 0.32857143 0.34285714 0.35714286 0.37142857 0.38571429 0.4 0.41428571 0.42857143 0.44285714 0.45714286 0.47142857 0.48571429 0.5 0.51428571 0.52857143 0.54285714 0.55714286 0.57142857 0.58571429 0.6 0.61428571 0.62857143 0.64285714 0.65714286 0.67142857 0.68571429 0.7 0.71428571 0.72857143 0.74285714 0.75714286 0.77142857 0.78571429 0.8 0.81428571 0.82857143 0.84285714 0.85714286 0.87142857 0.88571429 0.9 0.91428571 0.92857143 0.94285714 0.95714286 0.97142857 0.98571429 1 1 1 1 1 1
  arc A26 (11.0461, 7.2267) -> (10.2864, 8.2723) centre (0, 0) ccw
  spline S13 degree 5 poles (10.2864, 8.2723) (10.2763, 8.2722) (10.2561, 8.2721) (10.2259, 8.2717) (10.1857, 8.2711) (10.1356, 8.27) (10.0855, 8.2686) (10.0356, 8.2669) (9.9858, 8.2649) (9.9361, 8.2626) (9.8865, 8.26) (9.8371, 8.257) (9.7878, 8.2537) (9.7386, 8.2502) (9.6895, 8.2463) (9.6406, 8.242) (9.5918, 8.2375) (9.5431, 8.2327) (9.4946, 8.2275) (9.4463, 8.222) (9.398, 8.2162) (9.35, 8.2101) (9.302, 8.2037) (9.2543, 8.1969) (9.2067, 8.1898) (9.1592, 8.1824) (9.1119, 8.1746) (9.0648, 8.1666) (9.0179, 8.1582) (8.9711, 8.1495) (8.9245, 8.1404) (8.878, 8.131) (8.8318, 8.1213) (8.7858, 8.1113) (8.7399, 8.1009) (8.6942, 8.0902) (8.6487, 8.0791) (8.6035, 8.0677) (8.5584, 8.056) (8.5135, 8.0439) (8.4689, 8.0314) (8.4244, 8.0187) (8.3802, 8.0055) (8.3363, 7.992) (8.2925, 7.9781) (8.249, 7.9639) (8.2057, 7.9494) (8.1627, 7.9344) (8.1199, 7.9191) (8.0774, 7.9035) (8.0351, 7.8874) (7.9932, 7.871) (7.9515, 7.8541) (7.9101, 7.8369) (7.8691, 7.8192) (7.8283, 7.8011) (7.7879, 7.7826) (7.7476, 7.7638) (7.7077, 7.7447) (7.6682, 7.7251) (7.629, 7.7049) (7.5903, 7.6843) (7.5521, 7.663) (7.5144, 7.641) (7.4772, 7.6186) (7.4404, 7.5957) (7.4038, 7.5725) (7.3675, 7.549) (7.3316, 7.5252) (7.2964, 7.5006) (7.2623, 7.4748) (7.2362, 7.4528) (7.2174, 7.4354) (7.2053, 7.4233) (7.1993, 7.4172) knots -1 -1 -1 -1 -1 -1 -0.98571429 -0.97142857 -0.95714286 -0.94285714 -0.92857143 -0.91428571 -0.9 -0.88571429 -0.87142857 -0.85714286 -0.84285714 -0.82857143 -0.81428571 -0.8 -0.78571429 -0.77142857 -0.75714286 -0.74285714 -0.72857143 -0.71428571 -0.7 -0.68571429 -0.67142857 -0.65714286 -0.64285714 -0.62857143 -0.61428571 -0.6 -0.58571429 -0.57142857 -0.55714286 -0.54285714 -0.52857143 -0.51428571 -0.5 -0.48571429 -0.47142857 -0.45714286 -0.44285714 -0.42857143 -0.41428571 -0.4 -0.38571429 -0.37142857 -0.35714286 -0.34285714 -0.32857143 -0.31428571 -0.3 -0.28571429 -0.27142857 -0.25714286 -0.24285714 -0.22857143 -0.21428571 -0.2 -0.18571429 -0.17142857 -0.15714286 -0.14285714 -0.12857143 -0.11428571 -0.1 -0.08571429 -0.07142857 -0.05714286 -0.04285714 -0.02857143 -0.01428571 0 0 0 0 0 0
  line L13 (7.1993, 7.4172) -> (6.2867, 6.4785)
  arc A27 (5.273, 6.4217) -> (6.2867, 6.4785) centre (5.749, 7.0013) ccw
  arc A28 (5.273, 6.4217) -> (4.4779, 6.9993) centre (0, 0) ccw
  arc A29 (4.2187, 7.981) -> (4.4779, 6.9993) centre (4.8821, 7.6311) ccw
  line L14 (4.2187, 7.981) -> (4.8295, 9.139)
  spline S14 degree 5 poles (4.8295, 9.139) (4.8335, 9.1466) (4.8412, 9.1618) (4.8519, 9.185) (4.8648, 9.2167) (4.8788, 9.2571) (4.8913, 9.2982) (4.9029, 9.3397) (4.914, 9.3815) (4.9247, 9.4234) (4.9351, 9.4655) (4.945, 9.5079) (4.9542, 9.5505) (4.9626, 9.5934) (4.9704, 9.6366) (4.9774, 9.68) (4.9838, 9.7237) (4.9897, 9.7676) (4.9952, 9.8117) (5.0002, 9.8559) (5.0048, 9.9002) (5.0089, 9.9447) (5.0126, 9.9894) (5.0157, 10.0342) (5.0184, 10.0792) (5.0206, 10.1244) (5.0224, 10.1697) (5.0237, 10.2151) (5.0246, 10.2606) (5.0251, 10.3063) (5.0251, 10.352) (5.0248, 10.3979) (5.0241, 10.4439) (5.0229, 10.49) (5.0213, 10.5362) (5.0194, 10.5825) (5.017, 10.6289) (5.0142, 10.6754) (5.0111, 10.722) (5.0075, 10.7687) (5.0036, 10.8154) (4.9993, 10.8623) (4.9947, 10.9092) (4.9896, 10.9562) (4.9842, 11.0032) (4.9784, 11.0503) (4.9722, 11.0975) (4.9657, 11.1448) (4.9588, 11.1921) (4.9516, 11.2394) (4.9439, 11.2868) (4.936, 11.3343) (4.9277, 11.3818) (4.919, 11.4294) (4.9099, 11.477) (4.9006, 11.5247) (4.8908, 11.5724) (4.8807, 11.6201) (4.8703, 11.6679) (4.8595, 11.7157) (4.8484, 11.7635) (4.837, 11.8114) (4.8252, 11.8593) (4.8131, 11.9072) (4.8006, 11.9551) (4.7878, 12.0031) (4.7746, 12.0511) (4.7612, 12.099) (4.7473, 12.1471) (4.7332, 12.1951) (4.7187, 12.2431) (4.7069, 12.2815) (4.6979, 12.3104) (4.6918, 12.3296) (4.6887, 12.3392) knots 0 0 0 0 0 0 0.01428571 0.02857143 0.04285714 0.05714286 0.07142857 0.08571429 0.1 0.11428571 0.12857143 0.14285714 0.15714286 0.17142857 0.18571429 0.2 0.21428571 0.22857143 0.24285714 0.25714286 0.27142857 0.28571429 0.3 0.31428571 0.32857143 0.34285714 0.35714286 0.37142857 0.38571429 0.4 0.41428571 0.42857143 0.44285714 0.45714286 0.47142857 0.48571429 0.5 0.51428571 0.52857143 0.54285714 0.55714286 0.57142857 0.58571429 0.6 0.61428571 0.62857143 0.64285714 0.65714286 0.67142857 0.68571429 0.7 0.71428571 0.72857143 0.74285714 0.75714286 0.77142857 0.78571429 0.8 0.81428571 0.82857143 0.84285714 0.85714286 0.87142857 0.88571429 0.9 0.91428571 0.92857143 0.94285714 0.95714286 0.97142857 0.98571429 1 1 1 1 1 1
  arc A30 (4.6887, 12.3392) -> (3.4595, 12.7386) centre (0, 0) ccw
  spline S15 degree 5 poles (3.4595, 12.7386) (3.4514, 12.7326) (3.4352, 12.7206) (3.4109, 12.7026) (3.3788, 12.6785) (3.3388, 12.6481) (3.2992, 12.6176) (3.2598, 12.5869) (3.2207, 12.556) (3.1818, 12.5249) (3.1433, 12.4936) (3.105, 12.4621) (3.067, 12.4305) (3.0293, 12.3987) (2.9919, 12.3667) (2.9548, 12.3345) (2.918, 12.3022) (2.8815, 12.2697) (2.8453, 12.237) (2.8094, 12.2041) (2.7738, 12.1711) (2.7385, 12.1379) (2.7035, 12.1045) (2.6689, 12.0709) (2.6345, 12.0372) (2.6005, 12.0033) (2.5668, 11.9693) (2.5334, 11.9351) (2.5003, 11.9007) (2.4676, 11.8661) (2.4352, 11.8314) (2.4032, 11.7965) (2.3715, 11.7615) (2.3401, 11.7263) (2.3091, 11.6909) (2.2785, 11.6554) (2.2482, 11.6197) (2.2183, 11.5839) (2.1887, 11.5479) (2.1595, 11.5117) (2.1307, 11.4754) (2.1023, 11.439) (2.0742, 11.4024) (2.0466, 11.3656) (2.0194, 11.3287) (1.9925, 11.2916) (1.9661, 11.2544) (1.94, 11.217) (1.9144, 11.1795) (1.8892, 11.1418) (1.8644, 11.104) (1.8402, 11.066) (1.8164, 11.0279) (1.7931, 10.9896) (1.7702, 10.9512) (1.7479, 10.9126) (1.726, 10.8739) (1.7045, 10.835) (1.6835, 10.7961) (1.663, 10.7569) (1.6431, 10.7176) (1.624, 10.6782) (1.6056, 10.6385) (1.588, 10.5986) (1.5711, 10.5586) (1.5548, 10.5184) (1.5388, 10.4781) (1.5233, 10.4378) (1.5082, 10.3974) (1.4942, 10.3568) (1.4817, 10.3159) (1.4735, 10.2827) (1.4686, 10.2576) (1.4659, 10.2408) (1.4647, 10.2323) knots -1 -1 -1 -1 -1 -1 -0.98571429 -0.97142857 -0.95714286 -0.94285714 -0.92857143 -0.91428571 -0.9 -0.88571429 -0.87142857 -0.85714286 -0.84285714 -0.82857143 -0.81428571 -0.8 -0.78571429 -0.77142857 -0.75714286 -0.74285714 -0.72857143 -0.71428571 -0.7 -0.68571429 -0.67142857 -0.65714286 -0.64285714 -0.62857143 -0.61428571 -0.6 -0.58571429 -0.57142857 -0.55714286 -0.54285714 -0.52857143 -0.51428571 -0.5 -0.48571429 -0.47142857 -0.45714286 -0.44285714 -0.42857143 -0.41428571 -0.4 -0.38571429 -0.37142857 -0.35714286 -0.34285714 -0.32857143 -0.31428571 -0.3 -0.28571429 -0.27142857 -0.25714286 -0.24285714 -0.22857143 -0.21428571 -0.2 -0.18571429 -0.17142857 -0.15714286 -0.14285714 -0.12857143 -0.11428571 -0.1 -0.08571429 -0.07142857 -0.05714286 -0.04285714 -0.02857143 -0.01428571 0 0 0 0 0 0
  line L15 (1.4647, 10.2323) -> (1.2781, 8.9365)
  arc A31 (0.4914, 8.2947) -> (1.2781, 8.9365) centre (0.5357, 9.0433) ccw
  arc A32 (0.4914, 8.2947) -> (-0.4914, 8.2947) centre (0, 0) ccw
  arc A33 (-1.2781, 8.9365) -> (-0.4914, 8.2947) centre (-0.5357, 9.0433) ccw
  line L16 (-1.2781, 8.9365) -> (-1.4647, 10.2323)
  spline S16 degree 5 poles (-1.4647, 10.2323) (-1.4659, 10.2408) (-1.4686, 10.2576) (-1.4735, 10.2827) (-1.4817, 10.3159) (-1.4942, 10.3568) (-1.5082, 10.3974) (-1.5233, 10.4378) (-1.5388, 10.4781) (-1.5548, 10.5184) (-1.5711, 10.5586) (-1.588, 10.5986) (-1.6056, 10.6385) (-1.624, 10.6782) (-1.6431, 10.7176) (-1.663, 10.7569) (-1.6835, 10.7961) (-1.7045, 10.835) (-1.726, 10.8739) (-1.7479, 10.9126) (-1.7702, 10.9512) (-1.7931, 10.9896) (-1.8164, 11.0279) (-1.8402, 11.066) (-1.8644, 11.104) (-1.8892, 11.1418) (-1.9144, 11.1795) (-1.94, 11.217) (-1.9661, 11.2544) (-1.9925, 11.2916) (-2.0194, 11.3287) (-2.0466, 11.3656) (-2.0742, 11.4024) (-2.1023, 11.439) (-2.1307, 11.4754) (-2.1595, 11.5117) (-2.1887, 11.5479) (-2.2183, 11.5839) (-2.2482, 11.6197) (-2.2785, 11.6554) (-2.3091, 11.6909) (-2.3401, 11.7263) (-2.3715, 11.7615) (-2.4032, 11.7965) (-2.4352, 11.8314) (-2.4676, 11.8661) (-2.5003, 11.9007) (-2.5334, 11.9351) (-2.5668, 11.9693) (-2.6005, 12.0033) (-2.6345, 12.0372) (-2.6689, 12.0709) (-2.7035, 12.1045) (-2.7385, 12.1379) (-2.7738, 12.1711) (-2.8094, 12.2041) (-2.8453, 12.237) (-2.8815, 12.2697) (-2.918, 12.3022) (-2.9548, 12.3345) (-2.9919, 12.3667) (-3.0293, 12.3987) (-3.067, 12.4305) (-3.105, 12.4621) (-3.1433, 12.4936) (-3.1818, 12.5249) (-3.2207, 12.556) (-3.2598, 12.5869) (-3.2992, 12.6176) (-3.3388, 12.6481) (-3.3788, 12.6785) (-3.4109, 12.7026) (-3.4352, 12.7206) (-3.4514, 12.7326) (-3.4595, 12.7386) knots 0 0 0 0 0 0 0.01428571 0.02857143 0.04285714 0.05714286 0.07142857 0.08571429 0.1 0.11428571 0.12857143 0.14285714 0.15714286 0.17142857 0.18571429 0.2 0.21428571 0.22857143 0.24285714 0.25714286 0.27142857 0.28571429 0.3 0.31428571 0.32857143 0.34285714 0.35714286 0.37142857 0.38571429 0.4 0.41428571 0.42857143 0.44285714 0.45714286 0.47142857 0.48571429 0.5 0.51428571 0.52857143 0.54285714 0.55714286 0.57142857 0.58571429 0.6 0.61428571 0.62857143 0.64285714 0.65714286 0.67142857 0.68571429 0.7 0.71428571 0.72857143 0.74285714 0.75714286 0.77142857 0.78571429 0.8 0.81428571 0.82857143 0.84285714 0.85714286 0.87142857 0.88571429 0.9 0.91428571 0.92857143 0.94285714 0.95714286 0.97142857 0.98571429 1 1 1 1 1 1
  arc A34 (-3.4595, 12.7386) -> (-4.6887, 12.3392) centre (0, 0) ccw
  spline S17 degree 5 poles (-4.6887, 12.3392) (-4.6918, 12.3296) (-4.6979, 12.3104) (-4.7069, 12.2815) (-4.7187, 12.2431) (-4.7332, 12.1951) (-4.7473, 12.1471) (-4.7612, 12.099) (-4.7746, 12.0511) (-4.7878, 12.0031) (-4.8006, 11.9551) (-4.8131, 11.9072) (-4.8252, 11.8593) (-4.837, 11.8114) (-4.8484, 11.7635) (-4.8595, 11.7157) (-4.8703, 11.6679) (-4.8807, 11.6201) (-4.8908, 11.5724) (-4.9006, 11.5247) (-4.9099, 11.477) (-4.919, 11.4294) (-4.9277, 11.3818) (-4.936, 11.3343) (-4.9439, 11.2868) (-4.9516, 11.2394) (-4.9588, 11.1921) (-4.9657, 11.1448) (-4.9722, 11.0975) (-4.9784, 11.0503) (-4.9842, 11.0032) (-4.9896, 10.9562) (-4.9947, 10.9092) (-4.9993, 10.8623) (-5.0036, 10.8154) (-5.0075, 10.7687) (-5.0111, 10.722) (-5.0142, 10.6754) (-5.017, 10.6289) (-5.0194, 10.5825) (-5.0213, 10.5362) (-5.0229, 10.49) (-5.0241, 10.4439) (-5.0248, 10.3979) (-5.0251, 10.352) (-5.0251, 10.3063) (-5.0246, 10.2606) (-5.0237, 10.2151) (-5.0224, 10.1697) (-5.0206, 10.1244) (-5.0184, 10.0792) (-5.0157, 10.0342) (-5.0126, 9.9894) (-5.0089, 9.9447) (-5.0048, 9.9002) (-5.0002, 9.8559) (-4.9952, 9.8117) (-4.9897, 9.7676) (-4.9838, 9.7237) (-4.9774, 9.68) (-4.9704, 9.6366) (-4.9626, 9.5934) (-4.9542, 9.5505) (-4.945, 9.5079) (-4.9351, 9.4655) (-4.9247, 9.4234) (-4.914, 9.3815) (-4.9029, 9.3397) (-4.8913, 9.2982) (-4.8788, 9.2571) (-4.8648, 9.2167) (-4.8519, 9.185) (-4.8412, 9.1618) (-4.8335, 9.1466) (-4.8295, 9.139) knots -1 -1 -1 -1 -1 -1 -0.98571429 -0.97142857 -0.95714286 -0.94285714 -0.92857143 -0.91428571 -0.9 -0.88571429 -0.87142857 -0.85714286 -0.84285714 -0.82857143 -0.81428571 -0.8 -0.78571429 -0.77142857 -0.75714286 -0.74285714 -0.72857143 -0.71428571 -0.7 -0.68571429 -0.67142857 -0.65714286 -0.64285714 -0.62857143 -0.61428571 -0.6 -0.58571429 -0.57142857 -0.55714286 -0.54285714 -0.52857143 -0.51428571 -0.5 -0.48571429 -0.47142857 -0.45714286 -0.44285714 -0.42857143 -0.41428571 -0.4 -0.38571429 -0.37142857 -0.35714286 -0.34285714 -0.32857143 -0.31428571 -0.3 -0.28571429 -0.27142857 -0.25714286 -0.24285714 -0.22857143 -0.21428571 -0.2 -0.18571429 -0.17142857 -0.15714286 -0.14285714 -0.12857143 -0.11428571 -0.1 -0.08571429 -0.07142857 -0.05714286 -0.04285714 -0.02857143 -0.01428571 0 0 0 0 0 0
  line L17 (-4.8295, 9.139) -> (-4.2187, 7.981)
  arc A35 (-4.4779, 6.9993) -> (-4.2187, 7.981) centre (-4.8821, 7.6311) ccw
  arc A36 (-4.4779, 6.9993) -> (-5.273, 6.4217) centre (0, 0) ccw
  arc A37 (-6.2867, 6.4785) -> (-5.273, 6.4217) centre (-5.749, 7.0013) ccw
  line L18 (-6.2867, 6.4785) -> (-7.1993, 7.4172)